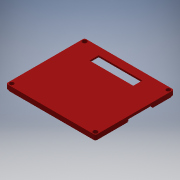
# Autodesk Inventor part: case rear
Saved by Autodesk Inventor 2018 (Build 220112000, 112)
## iProperties
Created: 2017-11-16
Part Number: case rear
Material: ABS-Kunststoff
Document SubType Name: Modeling
Designer: Till
Density: 1.06 g/cm^3
Appearance: Rot
Author: Till
Autodesk Inventor part; units mm, degrees
ref_plane "YZ Plane" through (0, 0, 0) normal (1, 0, 0) x (0, 1, 0)
ref_plane "XZ Plane" through (0, 0, 0) normal (0, 1, 0) x (-1, 0, 0)
ref_plane "XY Plane" through (0, 0, 0) normal (0, 0, 1) x (1, 0, 0)
sketch "Skizze1" plane through (0, 0, 0) normal (0, 0, 1) x (1, 0, 0)
  line L0 (52.3, 47.7) -> (-52.3, 47.7) projected
  arc A0 (-52.3, 47.7) -> (-54.3, 45.7) centre (-52.3, 45.7) ccw projected
  line L1 (54.3, 22.8) -> (54.3, 45.7) projected
  line L2 (-54.3, 45.7) -> (-54.3, -45.7) projected
  line L3 (-52.3, -47.7) -> (52.3, -47.7) projected
  arc A1 (-54.3, -45.7) -> (-52.3, -47.7) centre (-52.3, -45.7) ccw projected
  circle A2 centre (-50.8, -44.2) radius 1.5 projected
  circle A3 centre (50.8, 44.2) radius 1.5 projected
  arc A4 (52.3, -47.7) -> (54.3, -45.7) centre (52.3, -45.7) ccw projected
  line L4 (54.3, -45.7) -> (54.3, -8.2) projected
  line L5 (54.3, 22.8) -> (54.3, -8.2) projected
  arc A5 (54.3, 45.7) -> (52.3, 47.7) centre (52.3, 45.7) ccw projected
  circle A6 centre (-50.8, 44.2) radius 1.5 projected
  circle A7 centre (50.8, -44.2) radius 1.5 projected
  point P0 (0, 0)
extrude "Extrusion1" add sketch "Skizze1" along normal blind 7
sketch "Skizze2" plane through (0, 0, 0) normal (0, 0, -1) x (-1, 0, 0)
  line L0 (53.1, -44.5) -> (53.1, 44.5) projected
  line L1 (51.1, 46.5) -> (-51.1, 46.5) projected
  line L2 (-53.1, 44.5) -> (-53.1, -44.5) projected
  line L3 (-51.1, -46.5) -> (51.1, -46.5) projected
  line L4 (-51.3, -46.7) -> (51.3, -46.7)
  line L5 (53.3, -44.7) -> (53.3, 44.7)
  line L6 (51.3, 46.7) -> (-51.3, 46.7)
  line L7 (-53.3, 44.7) -> (-53.3, -44.7)
  line L8 (-53.3, -46.7) -> (53.3, 46.7) construction
  line L9 (53.3, -46.7) -> (-53.3, 46.7) construction
  arc A0 (53.3, 44.7) -> (51.3, 46.7) centre (51.3, 44.7) ccw
  arc A1 (-51.3, 46.7) -> (-53.3, 44.7) centre (-51.3, 44.7) ccw
  arc A2 (-53.3, -44.7) -> (-51.3, -46.7) centre (-51.3, -44.7) ccw
  arc A3 (51.3, -46.7) -> (53.3, -44.7) centre (51.3, -44.7) ccw
  line L10 (-56.7586, -49.6784) -> (56.7586, -49.6784)
  line L11 (56.7586, -49.6784) -> (56.7586, 49.6784)
  line L12 (56.7586, 49.6784) -> (-56.7586, 49.6784)
  line L13 (-56.7586, 49.6784) -> (-56.7586, -49.6784)
  line L14 (-56.7586, -49.6784) -> (56.7586, 49.6784) construction
  line L15 (56.7586, -49.6784) -> (-56.7586, 49.6784) construction
  point P0 (0, 0)
  dimension "d2" = 0.2
  dimension "d3" = 0.2
  dimension "d4" = 2
  constraints: 24 end point, 8 point on circle, 8 point on line, 8 tangent, 4 centre point, 4 midpoint, 4 parallel, 3 equal radius, 2 horizontal, 2 perpendicular
  measures "d2" distance between parallel lines of L1 L6
  measures "d3" distance between parallel lines of L0 L5
  measures "d4" radius of A0
extrude "Extrusion2" cut sketch "Skizze2" against normal blind 1.85
sketch "Skizze3" plane through (0, 0, 0) normal (0, 0, -1) x (-1, 0, 0)
  line L0 (-50.7142, 40.2858) -> (-46.8858, 44.1142)
  arc A0 (-45.4716, 44.7) -> (-46.8858, 44.1142) centre (-45.4716, 42.7) ccw
  line L1 (-45.4716, 44.7) -> (45.4716, 44.7)
  arc A1 (-50.7142, 40.2858) -> (-51.3, 38.8716) centre (-49.3, 38.8716) ccw
  line L2 (-51.3, -38.8716) -> (-51.3, 38.8716)
  line L3 (50.7142, -40.2858) -> (46.8858, -44.1142)
  arc A2 (50.7142, -40.2858) -> (51.3, -38.8716) centre (49.3, -38.8716) ccw
  line L4 (51.3, 38.8716) -> (51.3, -38.8716)
  arc A3 (45.4716, -44.7) -> (46.8858, -44.1142) centre (45.4716, -42.7) ccw
  line L5 (45.4716, -44.7) -> (-45.4716, -44.7)
  arc A4 (51.3, 38.8716) -> (50.7142, 40.2858) centre (49.3, 38.8716) ccw
  line L6 (46.8858, 44.1142) -> (50.7142, 40.2858)
  arc A5 (46.8858, 44.1142) -> (45.4716, 44.7) centre (45.4716, 42.7) ccw
  arc A6 (-46.8858, -44.1142) -> (-45.4716, -44.7) centre (-45.4716, -42.7) ccw
  line L7 (-46.8858, -44.1142) -> (-50.7142, -40.2858)
  arc A7 (-51.3, -38.8716) -> (-50.7142, -40.2858) centre (-49.3, -38.8716) ccw
  circle A8 centre (-50.8, -44.2) radius 1.5
  circle A9 centre (-50.8, 44.2) radius 1.5
  circle A10 centre (50.8, 44.2) radius 1.5
  circle A11 centre (50.8, -44.2) radius 1.5
  point P0 (0, 0)
  constraints: 16 end point, 16 point on circle, 12 centre point
extrude "Extrusion3" cut sketch "Skizze3" against normal blind 5 contours L0 A0 L1 A5 L6 A4 L4 A2 L3 A3 L5 A6 L7 A7 L2 A1
sketch "Skizze4" plane through (54.3, -45.7, 7) normal (1, 0, 0) x (0, 0, -1)
  line L0 (3.15, 38) -> (3.15, 68.5)
  line L1 (0, 0) -> (0, 91.4) projected
  line L2 (7, 90.4) -> (7, 1) projected
  line L3 (5.15, -2) -> (0, -2) projected
  line L4 (3.15, 68.5) -> (7, 68.5)
  line L5 (7, 1) -> (7, 90.4) projected
  line L6 (3.15, 38) -> (7, 38)
  line L7 (7, 68.5) -> (7, 38)
  point P0 (7, 45.7)
  dimension "d11" = 3.85
  dimension "d13" = 30.5
  dimension "d14" = 40
  constraints: 8 end point, 2 point on line, 1 collinear, 1 parallel, 1 perpendicular, 1 vertical
  measures "d11" distance between parallel lines of L2 L0
  measures "d13" distance of L0.start L0.end
  measures "d14" distance between parallel lines of L3 L6
extrude "Extrusion4" cut sketch "Skizze4" against normal up to next
sketch "Skizze5" plane through (0, 0, 7) normal (0, 0, 1) x (1, 0, 0)
  circle A0 centre (-50.8, 44.2) radius 1.5 projected
  circle A1 centre (-50.8, 44.2) radius 2.7
  line L0 (52.3, 47.7) -> (-52.3, 47.7) projected
  circle A2 centre (50.8, 44.2) radius 1.5 projected
  circle A3 centre (50.8, 44.2) radius 2.5
  line L1 (-51.3, 46.7) -> (51.3, 46.7) projected
  circle A4 centre (50.8, -44.2) radius 1.5 projected
  circle A5 centre (50.8, -44.2) radius 2.7
  line L2 (54.3, -45.7) -> (54.3, 45.7) projected
  circle A6 centre (-50.8, -44.2) radius 1.5 projected
  circle A7 centre (-50.8, -44.2) radius 2.5
  line L3 (51.3, -46.7) -> (-51.3, -46.7) projected
  point P0 (0, 0)
  dimension "d17" = 0.8
  dimension "d18" = 0.8
  constraints: 4 centre point, 4 coincident, 2 tangent
  measures "d17" distance edge to line of A1 L0
  measures "d18" distance edge to line of A5 L2
extrude "Extrusion5" cut sketch "Skizze5" against normal blind 4
sketch "Skizze6" plane through (0, 0, 7) normal (0, 0, 1) x (1, 0, 0)
  line L0 (-27.7, 38.2) -> (25.3, 38.2)
  line L1 (25.3, 38.2) -> (25.3, 27.2)
  line L2 (25.3, 27.2) -> (-27.7, 27.2)
  line L3 (-27.7, 27.2) -> (-27.7, 38.2)
  line L4 (54.3, -45.7) -> (54.3, 45.7) projected
  line L5 (52.3, 47.7) -> (-52.3, 47.7) projected
  point P0 (0, 0)
  dimension "d21" = 53
  dimension "d22" = 11
  dimension "d23" = 29
  dimension "d24" = 9.5
  constraints: 8 end point, 2 parallel, 1 horizontal, 1 perpendicular
  measures "d21" distance of L0.start L0.end
  measures "d22" distance of L0.end L1.end
  measures "d23" distance between parallel lines of L4 L1
  measures "d24" distance between parallel lines of L5 L0
extrude "Extrusion6" cut sketch "Skizze6" against normal up to next
